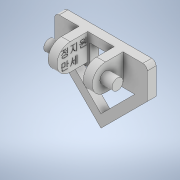
# Autodesk Inventor part: 02-2
Saved by Autodesk Inventor 2022 (Build 260153000, 153)
## iProperties
Created: 2021-09-12
Part Number: 02-2
Material: 일반
Document SubType Name: Modeling
Designer: 서울공업고등학교
Density: 1 g/cm^3
Appearance: 기본값
Author: 서울공업고등학교
Autodesk Inventor part; units mm, degrees
ref_plane "XZ Plane" through (0, 0, 0) normal (0, 1, 0) x (-1, 0, 0)
ref_plane "XY Plane" through (0, 0, 0) normal (0, 0, 1) x (1, 0, 0)
sketch "스케치1" plane through (0, 0, 0) normal (0, 0, 1) x (1, 0, 0)
  line L0 (0, 0) -> (0, 50)
  line L1 (0, 0) -> (50, 0) construction
  line L2 (0, 0) -> (-21, 21)
  line L3 (-21, 21) -> (-21, 35)
  line L4 (-21, 35) -> (0, 35)
  line L5 (0, 5.6569) -> (-15.3431, 21)
  line L6 (-15.3431, 21) -> (-5, 21)
  line L7 (-5, 21) -> (-5, 31)
  line L8 (-5, 31) -> (0, 31)
  line L9 (0, 0) -> (21, 21)
  line L10 (21, 21) -> (21, 35)
  line L11 (21, 35) -> (0, 35)
  line L12 (0, 5.6569) -> (15.3431, 21)
  line L13 (15.3431, 21) -> (5, 21)
  line L14 (5, 21) -> (5, 31)
  line L15 (5, 31) -> (0, 31)
  dimension "d0" = 50
  dimension "d2" = 35
  dimension "d3" = 45
  dimension "d4" = 4
  dimension "d5" = 10
  dimension "d6" = 42
  dimension "d7" = 10
  dimension "d8" = 4
  constraints: 32 end point, 5 symmetric about line, 4 perpendicular, 3 point on line, 2 parallel, 2 vertical, 1 horizontal
  measures "d0" distance of L0.start L0.end
  measures "d2" distance from line of L4 L0.start
  measures "d3" angle of L0 L2
  measures "d4" distance between parallel lines of L4 L8
  measures "d5" distance between parallel lines of L6 L8
  measures "d6" diameter of L3 L0
  measures "d7" diameter of L7 L0
  measures "d8" distance between parallel lines of L2 L5
extrude "돌출1" add sketch "스케치1" against normal blind 4 contours L2 L3 L4 L0 L8 L7 L6 L5 | L0 L12 L13 L14 L15 L11 L10 L9
ref_plane "작업 평면1" through (6, 0, 0) normal (1, 0, 0) x (0, 1, 0)
sketch "스케치2" plane through (6, 0, 0) normal (1, 0, 0) x (0, 1, 0)
  arc A0 (35, 8) -> (23, 8) centre (29, 8) ccw
  circle A1 centre (29, 8) radius 2.5
  line L0 (35, 0) -> (21, 0) projected
  line L1 (35, 0) -> (35, 8)
  line L2 (23, 8) -> (23, 0)
  line L3 (21, -4) -> (35, -4) projected
  point P0 (0, 0)
  dimension "d12" = 12
  dimension "d13" = 5
  dimension "d14" = 12
  dimension "d15" = 18
  dimension "d16" = 12
  constraints: 4 end point, 3 point on circle, 2 centre point, 2 point on line, 1 coincident, 1 parallel, 1 tangent, 1 vertical
  measures "d12" diameter of A0
  measures "d13" diameter of A1
  measures "d14" distance from line of L3 A0.centre
  measures "d16" distance between parallel lines of L2 L1
extrude "돌출2" add sketch "스케치2" along normal blind 4
extrude "돌출3" add sketch "스케치2" along normal blind 9.5 contours A1
mirror "미러1" about plane through (0, 0, 0) normal (1, 0, 0) of "돌출2", "돌출3"
fillet "모깎기1" radius 2 2 edges at (21, 35, -2) (-21, 35, -2)
sketch "스케치3" plane through (-6, 29, 8) normal (1, 0, 0) x (0, 0, -1)
  line L0 (-4.519, 4.2774) -> (7.7198, 4.2774) construction
  line L1 (7.7198, 4.2774) -> (7.7198, -3.1581) construction
  line L2 (7.7198, -3.1581) -> (-4.519, -3.1581) construction
  line L3 (-4.519, -3.1581) -> (-4.519, 4.2774) construction
  spline S0 degree 2 poles (-2.422, 2.0914) (-3.0938, 2.0914) (-3.452, 1.9062) knots 0 0 0 1 1 1
  spline S1 degree 2 poles (-3.452, 1.9062) (-3.7706, 1.7432) (-3.7706, 1.4616) knots 0 0 0 1 1 1
  spline S2 degree 2 poles (-3.7706, 1.4616) (-3.7706, 1.1899) (-3.452, 1.0268) knots 0 0 0 1 1 1
  spline S3 degree 2 poles (-3.452, 1.0268) (-3.0938, 0.8416) (-2.422, 0.8416) knots 0 0 0 1 1 1
  spline S4 degree 2 poles (-2.422, 0.8416) (-1.7526, 0.8416) (-1.3994, 1.0268) knots 0 0 0 1 1 1
  spline S5 degree 2 poles (-1.3994, 1.0268) (-1.0758, 1.1899) (-1.0758, 1.4616) knots 0 0 0 1 1 1
  spline S6 degree 2 poles (-1.0758, 1.4616) (-1.0758, 1.7432) (-1.3994, 1.9062) knots 0 0 0 1 1 1
  spline S7 degree 2 poles (-1.3994, 1.9062) (-1.7526, 2.0914) (-2.422, 2.0914) knots 0 0 0 1 1 1
  spline S8 degree 2 poles (-2.422, 1.879) (-1.8662, 1.879) (-1.5797, 1.7654) knots 0 0 0 1 1 1
  spline S9 degree 2 poles (-1.5797, 1.7654) (-1.3129, 1.6542) (-1.3129, 1.4616) knots 0 0 0 1 1 1
  spline S10 degree 2 poles (-1.3129, 1.4616) (-1.3129, 1.2763) (-1.5797, 1.1701) knots 0 0 0 1 1 1
  spline S11 degree 2 poles (-1.5797, 1.1701) (-1.8662, 1.0515) (-2.422, 1.0515) knots 0 0 0 1 1 1
  spline S12 degree 2 poles (-2.422, 1.0515) (-2.9851, 1.0515) (-3.2717, 1.1701) knots 0 0 0 1 1 1
  spline S13 degree 2 poles (-3.2717, 1.1701) (-3.5335, 1.2763) (-3.5335, 1.4616) knots 0 0 0 1 1 1
  spline S14 degree 2 poles (-3.5335, 1.4616) (-3.5335, 1.6542) (-3.2717, 1.7654) knots 0 0 0 1 1 1
  spline S15 degree 2 poles (-3.2717, 1.7654) (-2.9851, 1.879) (-2.422, 1.879) knots 0 0 0 1 1 1
  line L4 (-1.9774, 4.1786) -> (-3.8348, 4.1786)
  spline S16 degree 2 poles (-3.8348, 4.1786) (-3.9509, 4.1786) (-3.9509, 4.0748) knots 0 0 0 1 1 1
  spline S17 degree 2 poles (-3.9509, 4.0748) (-3.9559, 3.9686) (-3.8398, 3.9686) knots 0 0 0 1 1 1
  line L5 (-3.8398, 3.9686) -> (-3.0296, 3.9686)
  line L6 (-3.0296, 3.9686) -> (-3.0296, 3.8328)
  spline S18 degree 2 poles (-3.0296, 3.8328) (-3.0296, 3.403) (-3.3112, 3.0967) knots 0 0 0 1 1 1
  spline S19 degree 2 poles (-3.3112, 3.0967) (-3.5458, 2.8423) (-3.983, 2.662) knots 0 0 0 1 1 1
  spline S20 degree 2 poles (-3.983, 2.662) (-4.0374, 2.6422) (-4.0522, 2.5978) knots 0 0 0 1 1 1
  spline S21 degree 2 poles (-4.0522, 2.5978) (-4.0645, 2.5558) (-4.0448, 2.5138) knots 0 0 0 1 1 1
  spline S22 degree 2 poles (-4.0448, 2.5138) (-4.0201, 2.4693) (-3.9781, 2.4545) knots 0 0 0 1 1 1
  spline S23 degree 2 poles (-3.9781, 2.4545) (-3.9336, 2.4323) (-3.8818, 2.4496) knots 0 0 0 1 1 1
  spline S24 degree 2 poles (-3.8818, 2.4496) (-3.5137, 2.5928) (-3.2544, 2.8324) knots 0 0 0 1 1 1
  spline S25 degree 2 poles (-3.2544, 2.8324) (-3.0049, 3.0696) (-2.911, 3.3437) knots 0 0 0 1 1 1
  spline S26 degree 2 poles (-2.911, 3.3437) (-2.8419, 3.1017) (-2.5578, 2.8547) knots 0 0 0 1 1 1
  spline S27 degree 2 poles (-2.5578, 2.8547) (-2.296, 2.6299) (-1.9601, 2.4866) knots 0 0 0 1 1 1
  spline S28 degree 2 poles (-1.9601, 2.4866) (-1.9033, 2.4619) (-1.8489, 2.4792) knots 0 0 0 1 1 1
  spline S29 degree 2 poles (-1.8489, 2.4792) (-1.802, 2.4965) (-1.7773, 2.541) knots 0 0 0 1 1 1
  spline S30 degree 2 poles (-1.7773, 2.541) (-1.7551, 2.5854) (-1.7674, 2.6299) knots 0 0 0 1 1 1
  spline S31 degree 2 poles (-1.7674, 2.6299) (-1.7847, 2.6768) (-1.8391, 2.6966) knots 0 0 0 1 1 1
  spline S32 degree 2 poles (-1.8391, 2.6966) (-2.2466, 2.8596) (-2.4837, 3.1066) knots 0 0 0 1 1 1
  spline S33 degree 2 poles (-2.4837, 3.1066) (-2.7875, 3.4154) (-2.7875, 3.8427) knots 0 0 0 1 1 1
  line L7 (-2.7875, 3.8427) -> (-2.7875, 3.9686)
  line L8 (-2.7875, 3.9686) -> (-1.9774, 3.9686)
  spline S34 degree 2 poles (-1.9774, 3.9686) (-1.8736, 3.9686) (-1.8736, 4.0748) knots 0 0 0 1 1 1
  spline S35 degree 2 poles (-1.8736, 4.0748) (-1.8736, 4.1786) (-1.9774, 4.1786) knots 0 0 0 1 1 1
  line L9 (-1.1055, 2.2866) -> (-1.1055, 4.1588)
  spline S36 degree 2 poles (-1.1055, 4.1588) (-1.1055, 4.2156) (-1.145, 4.2478) knots 0 0 0 1 1 1
  spline S37 degree 2 poles (-1.145, 4.2478) (-1.1796, 4.2774) (-1.2265, 4.2774) knots 0 0 0 1 1 1
  spline S38 degree 2 poles (-1.2265, 4.2774) (-1.2808, 4.2774) (-1.3129, 4.2453) knots 0 0 0 1 1 1
  spline S39 degree 2 poles (-1.3129, 4.2453) (-1.35, 4.2107) (-1.35, 4.1539) knots 0 0 0 1 1 1
  line L10 (-1.35, 4.1539) -> (-1.35, 3.4425)
  line L11 (-1.35, 3.4425) -> (-2.0515, 3.4425)
  spline S40 degree 2 poles (-2.0515, 3.4425) (-2.1083, 3.4425) (-2.1355, 3.4129) knots 0 0 0 1 1 1
  spline S41 degree 2 poles (-2.1355, 3.4129) (-2.1651, 3.3808) (-2.1651, 3.3388) knots 0 0 0 1 1 1
  spline S42 degree 2 poles (-2.1651, 3.3388) (-2.1602, 3.2993) (-2.128, 3.2647) knots 0 0 0 1 1 1
  spline S43 degree 2 poles (-2.128, 3.2647) (-2.091, 3.2326) (-2.0292, 3.2326) knots 0 0 0 1 1 1
  line L12 (-2.0292, 3.2326) -> (-1.35, 3.2326)
  line L13 (-1.35, 3.2326) -> (-1.35, 2.2866)
  spline S44 degree 2 poles (-1.35, 2.2866) (-1.35, 2.2248) (-1.3129, 2.1878) knots 0 0 0 1 1 1
  spline S45 degree 2 poles (-1.3129, 2.1878) (-1.2808, 2.1556) (-1.2265, 2.1556) knots 0 0 0 1 1 1
  spline S46 degree 2 poles (-1.2265, 2.1556) (-1.1796, 2.1556) (-1.145, 2.1878) knots 0 0 0 1 1 1
  spline S47 degree 2 poles (-1.145, 2.1878) (-1.1055, 2.2248) (-1.1055, 2.2866) knots 0 0 0 1 1 1
  line L14 (2.2142, 4.149) -> (0.3568, 4.149)
  spline S48 degree 2 poles (0.3568, 4.149) (0.2407, 4.149) (0.2407, 4.0452) knots 0 0 0 1 1 1
  spline S49 degree 2 poles (0.2407, 4.0452) (0.2358, 3.939) (0.3519, 3.939) knots 0 0 0 1 1 1
  line L15 (0.3519, 3.939) -> (1.162, 3.939)
  line L16 (1.162, 3.939) -> (1.162, 3.2721)
  spline S50 degree 2 poles (1.162, 3.2721) (1.162, 2.6324) (0.8878, 2.1062) knots 0 0 0 1 1 1
  spline S51 degree 2 poles (0.8878, 2.1062) (0.626, 1.59) (0.2135, 1.3776) knots 0 0 0 1 1 1
  spline S52 degree 2 poles (0.2135, 1.3776) (0.1592, 1.3529) (0.1419, 1.3035) knots 0 0 0 1 1 1
  spline S53 degree 2 poles (0.1419, 1.3035) (0.1296, 1.259) (0.1543, 1.2121) knots 0 0 0 1 1 1
  spline S54 degree 2 poles (0.1543, 1.2121) (0.1765, 1.1726) (0.216, 1.1553) knots 0 0 0 1 1 1
  spline S55 degree 2 poles (0.216, 1.1553) (0.2605, 1.1355) (0.3099, 1.1602) knots 0 0 0 1 1 1
  spline S56 degree 2 poles (0.3099, 1.1602) (0.6557, 1.3307) (0.9298, 1.7357) knots 0 0 0 1 1 1
  spline S57 degree 2 poles (0.9298, 1.7357) (1.1991, 2.1334) (1.2806, 2.5632) knots 0 0 0 1 1 1
  spline S58 degree 2 poles (1.2806, 2.5632) (1.3497, 2.1458) (1.6289, 1.7357) knots 0 0 0 1 1 1
  spline S59 degree 2 poles (1.6289, 1.7357) (1.908, 1.3356) (2.234, 1.1602) knots 0 0 0 1 1 1
  spline S60 degree 2 poles (2.234, 1.1602) (2.2958, 1.1257) (2.3501, 1.1429) knots 0 0 0 1 1 1
  spline S61 degree 2 poles (2.3501, 1.1429) (2.3995, 1.1553) (2.4242, 1.1998) knots 0 0 0 1 1 1
  spline S62 degree 2 poles (2.4242, 1.1998) (2.444, 1.2417) (2.4316, 1.2911) knots 0 0 0 1 1 1
  spline S63 degree 2 poles (2.4316, 1.2911) (2.4193, 1.3405) (2.3649, 1.3677) knots 0 0 0 1 1 1
  spline S64 degree 2 poles (2.3649, 1.3677) (1.9351, 1.6048) (1.6733, 2.1137) knots 0 0 0 1 1 1
  spline S65 degree 2 poles (1.6733, 2.1137) (1.4041, 2.6373) (1.4041, 3.277) knots 0 0 0 1 1 1
  line L17 (1.4041, 3.277) -> (1.4041, 3.939)
  line L18 (1.4041, 3.939) -> (2.2142, 3.939)
  spline S66 degree 2 poles (2.2142, 3.939) (2.318, 3.939) (2.318, 4.0452) knots 0 0 0 1 1 1
  spline S67 degree 2 poles (2.318, 4.0452) (2.318, 4.149) (2.2142, 4.149) knots 0 0 0 1 1 1
  line L19 (3.0862, 0.975) -> (3.0862, 4.1613)
  spline S68 degree 2 poles (3.0862, 4.1613) (3.0862, 4.2156) (3.0466, 4.2478) knots 0 0 0 1 1 1
  spline S69 degree 2 poles (3.0466, 4.2478) (3.0121, 4.2725) (2.9651, 4.2725) knots 0 0 0 1 1 1
  spline S70 degree 2 poles (2.9651, 4.2725) (2.9108, 4.2725) (2.8787, 4.2478) knots 0 0 0 1 1 1
  spline S71 degree 2 poles (2.8787, 4.2478) (2.8416, 4.2156) (2.8416, 4.1613) knots 0 0 0 1 1 1
  line L20 (2.8416, 4.1613) -> (2.8416, 0.975)
  spline S72 degree 2 poles (2.8416, 0.975) (2.8416, 0.9182) (2.8787, 0.8811) knots 0 0 0 1 1 1
  spline S73 degree 2 poles (2.8787, 0.8811) (2.9108, 0.849) (2.9651, 0.849) knots 0 0 0 1 1 1
  spline S74 degree 2 poles (2.9651, 0.849) (3.0121, 0.849) (3.0466, 0.8811) knots 0 0 0 1 1 1
  spline S75 degree 2 poles (3.0466, 0.8811) (3.0862, 0.9182) (3.0862, 0.975) knots 0 0 0 1 1 1
  spline S76 degree 2 poles (5.5068, 4.1934) (4.9807, 4.1934) (4.6892, 4.0082) knots 0 0 0 1 1 1
  spline S77 degree 2 poles (4.6892, 4.0082) (4.4323, 3.8451) (4.4323, 3.5957) knots 0 0 0 1 1 1
  spline S78 degree 2 poles (4.4323, 3.5957) (4.4323, 3.3511) (4.6892, 3.1881) knots 0 0 0 1 1 1
  spline S79 degree 2 poles (4.6892, 3.1881) (4.9807, 3.0029) (5.5068, 3.0029) knots 0 0 0 1 1 1
  spline S80 degree 2 poles (5.5068, 3.0029) (6.0255, 3.0029) (6.3169, 3.1881) knots 0 0 0 1 1 1
  spline S81 degree 2 poles (6.3169, 3.1881) (6.5788, 3.3511) (6.5788, 3.5957) knots 0 0 0 1 1 1
  spline S82 degree 2 poles (6.5788, 3.5957) (6.5788, 3.8451) (6.3169, 4.0082) knots 0 0 0 1 1 1
  spline S83 degree 2 poles (6.3169, 4.0082) (6.0255, 4.1934) (5.5068, 4.1934) knots 0 0 0 1 1 1
  spline S84 degree 2 poles (5.5068, 3.9835) (5.9193, 3.9835) (6.1391, 3.8649) knots 0 0 0 1 1 1
  spline S85 degree 2 poles (6.1391, 3.8649) (6.3367, 3.7587) (6.3367, 3.5957) knots 0 0 0 1 1 1
  spline S86 degree 2 poles (6.3367, 3.5957) (6.3367, 3.4376) (6.1391, 3.3314) knots 0 0 0 1 1 1
  spline S87 degree 2 poles (6.1391, 3.3314) (5.9193, 3.2128) (5.5068, 3.2128) knots 0 0 0 1 1 1
  spline S88 degree 2 poles (5.5068, 3.2128) (5.0869, 3.2128) (4.867, 3.3314) knots 0 0 0 1 1 1
  spline S89 degree 2 poles (4.867, 3.3314) (4.6744, 3.4376) (4.6744, 3.5957) knots 0 0 0 1 1 1
  spline S90 degree 2 poles (4.6744, 3.5957) (4.6744, 3.7587) (4.867, 3.8649) knots 0 0 0 1 1 1
  spline S91 degree 2 poles (4.867, 3.8649) (5.0869, 3.9835) (5.5068, 3.9835) knots 0 0 0 1 1 1
  line L21 (7.2778, 1.8444) -> (7.2778, 4.1662)
  spline S92 degree 2 poles (7.2778, 4.1662) (7.2778, 4.2206) (7.2383, 4.2478) knots 0 0 0 1 1 1
  spline S93 degree 2 poles (7.2383, 4.2478) (7.2037, 4.2774) (7.1567, 4.2774) knots 0 0 0 1 1 1
  spline S94 degree 2 poles (7.1567, 4.2774) (7.1024, 4.2774) (7.0703, 4.2478) knots 0 0 0 1 1 1
  spline S95 degree 2 poles (7.0703, 4.2478) (7.0332, 4.2156) (7.0332, 4.1638) knots 0 0 0 1 1 1
  line L22 (7.0332, 4.1638) -> (7.0332, 2.3656)
  line L23 (7.0332, 2.3656) -> (6.2206, 2.3656)
  spline S96 degree 2 poles (6.2206, 2.3656) (6.1638, 2.3656) (6.1317, 2.336) knots 0 0 0 1 1 1
  spline S97 degree 2 poles (6.1317, 2.336) (6.1021, 2.3088) (6.107, 2.2643) knots 0 0 0 1 1 1
  spline S98 degree 2 poles (6.107, 2.2643) (6.107, 2.2223) (6.144, 2.1927) knots 0 0 0 1 1 1
  spline S99 degree 2 poles (6.144, 2.1927) (6.1811, 2.1606) (6.2453, 2.1606) knots 0 0 0 1 1 1
  line L24 (6.2453, 2.1606) -> (7.0332, 2.1606)
  line L25 (7.0332, 2.1606) -> (7.0332, 1.8444)
  spline S100 degree 2 poles (7.0332, 1.8444) (7.0332, 1.7876) (7.0703, 1.7506) knots 0 0 0 1 1 1
  spline S101 degree 2 poles (7.0703, 1.7506) (7.1024, 1.7209) (7.1567, 1.7209) knots 0 0 0 1 1 1
  spline S102 degree 2 poles (7.1567, 1.7209) (7.2037, 1.7209) (7.2383, 1.7506) knots 0 0 0 1 1 1
  spline S103 degree 2 poles (7.2383, 1.7506) (7.2778, 1.7876) (7.2778, 1.8444) knots 0 0 0 1 1 1
  spline S104 degree 2 poles (4.8868, 1.8271) (4.8868, 1.8864) (4.8473, 1.9185) knots 0 0 0 1 1 1
  spline S105 degree 2 poles (4.8473, 1.9185) (4.8127, 1.9506) (4.7658, 1.9506) knots 0 0 0 1 1 1
  spline S106 degree 2 poles (4.7658, 1.9506) (4.7114, 1.9506) (4.6793, 1.9185) knots 0 0 0 1 1 1
  spline S107 degree 2 poles (4.6793, 1.9185) (4.6423, 1.8839) (4.6423, 1.8271) knots 0 0 0 1 1 1
  line L26 (4.6423, 1.8271) -> (4.6423, 1.3109)
  spline S108 degree 2 poles (4.6423, 1.3109) (4.6423, 1.1528) (4.7534, 1.0491) knots 0 0 0 1 1 1
  spline S109 degree 2 poles (4.7534, 1.0491) (4.8646, 0.9478) (5.0301, 0.9478) knots 0 0 0 1 1 1
  line L27 (5.0301, 0.9478) -> (7.3074, 0.9478)
  spline S110 degree 2 poles (7.3074, 0.9478) (7.4136, 0.9478) (7.4136, 1.054) knots 0 0 0 1 1 1
  spline S111 degree 2 poles (7.4136, 1.054) (7.4136, 1.1578) (7.3074, 1.1578) knots 0 0 0 1 1 1
  line L28 (7.3074, 1.1578) -> (5.0869, 1.1578)
  spline S112 degree 2 poles (5.0869, 1.1578) (4.9683, 1.1578) (4.9288, 1.1948) knots 0 0 0 1 1 1
  spline S113 degree 2 poles (4.9288, 1.1948) (4.8868, 1.2343) (4.8868, 1.3455) knots 0 0 0 1 1 1
  line L29 (4.8868, 1.3455) -> (4.8868, 1.8271)
  line L30 (5.366, 2.5286) -> (5.366, 2.3483)
  spline S114 degree 2 poles (5.366, 2.3483) (5.366, 2.2372) (5.3413, 2.1482) knots 0 0 0 1 1 1
  spline S115 degree 2 poles (5.3413, 2.1482) (5.3166, 2.0568) (5.2795, 1.9926) knots 0 0 0 1 1 1
  spline S116 degree 2 poles (5.2795, 1.9926) (5.2104, 1.9012) (5.2919, 1.842) knots 0 0 0 1 1 1
  spline S117 degree 2 poles (5.2919, 1.842) (5.3734, 1.7753) (5.4475, 1.8568) knots 0 0 0 1 1 1
  spline S118 degree 2 poles (5.4475, 1.8568) (5.5167, 1.9432) (5.5611, 2.0815) knots 0 0 0 1 1 1
  spline S119 degree 2 poles (5.5611, 2.0815) (5.6105, 2.2248) (5.6105, 2.3779) knots 0 0 0 1 1 1
  line L31 (5.6105, 2.3779) -> (5.6105, 2.541)
  line L32 (5.6105, 2.541) -> (6.6183, 2.5706)
  spline S120 degree 2 poles (6.6183, 2.5706) (6.6677, 2.5755) (6.6998, 2.6126) knots 0 0 0 1 1 1
  spline S121 degree 2 poles (6.6998, 2.6126) (6.7245, 2.6398) (6.7245, 2.6818) knots 0 0 0 1 1 1
  spline S122 degree 2 poles (6.7245, 2.6818) (6.7196, 2.7262) (6.6874, 2.7509) knots 0 0 0 1 1 1
  spline S123 degree 2 poles (6.6874, 2.7509) (6.6504, 2.7781) (6.5936, 2.7707) knots 0 0 0 1 1 1
  spline S124 degree 2 poles (6.5936, 2.7707) (6.2132, 2.7509) (5.5265, 2.7336) knots 0 0 0 1 1 1
  spline S125 degree 2 poles (5.5265, 2.7336) (4.8819, 2.7163) (4.3187, 2.7163) knots 0 0 0 1 1 1
  spline S126 degree 2 poles (4.3187, 2.7163) (4.2125, 2.7163) (4.2075, 2.6175) knots 0 0 0 1 1 1
  spline S127 degree 2 poles (4.2075, 2.6175) (4.2026, 2.5163) (4.3063, 2.5163) knots 0 0 0 1 1 1
  line L33 (4.3063, 2.5163) -> (5.366, 2.5286)
  line L34 (-2.6171, -0.8695) -> (-3.5878, -0.8695)
  spline S128 degree 2 poles (-3.5878, -0.8695) (-3.7533, -0.8695) (-3.8571, -0.9757) knots 0 0 0 1 1 1
  spline S129 degree 2 poles (-3.8571, -0.9757) (-3.9509, -1.0745) (-3.9509, -1.2227) knots 0 0 0 1 1 1
  line L35 (-3.9509, -1.2227) -> (-3.9509, -2.3565)
  spline S130 degree 2 poles (-3.9509, -2.3565) (-3.9509, -2.5047) (-3.862, -2.5985) knots 0 0 0 1 1 1
  spline S131 degree 2 poles (-3.862, -2.5985) (-3.7657, -2.6924) (-3.615, -2.6924) knots 0 0 0 1 1 1
  line L36 (-3.615, -2.6924) -> (-2.6048, -2.6924)
  spline S132 degree 2 poles (-2.6048, -2.6924) (-2.4368, -2.6924) (-2.3331, -2.6035) knots 0 0 0 1 1 1
  spline S133 degree 2 poles (-2.3331, -2.6035) (-2.2318, -2.5121) (-2.2318, -2.3515) knots 0 0 0 1 1 1
  line L37 (-2.2318, -2.3515) -> (-2.2318, -1.1931)
  spline S134 degree 2 poles (-2.2318, -1.1931) (-2.2318, -1.0548) (-2.338, -0.9634) knots 0 0 0 1 1 1
  spline S135 degree 2 poles (-2.338, -0.9634) (-2.4442, -0.8695) (-2.6171, -0.8695) knots 0 0 0 1 1 1
  line L38 (-2.4689, -1.2548) -> (-2.4689, -2.3268)
  spline S136 degree 2 poles (-2.4689, -2.3268) (-2.4689, -2.4157) (-2.5134, -2.4528) knots 0 0 0 1 1 1
  spline S137 degree 2 poles (-2.5134, -2.4528) (-2.5554, -2.4824) (-2.6542, -2.4824) knots 0 0 0 1 1 1
  line L39 (-2.6542, -2.4824) -> (-3.5285, -2.4824)
  spline S138 degree 2 poles (-3.5285, -2.4824) (-3.6323, -2.4824) (-3.6669, -2.4503) knots 0 0 0 1 1 1
  spline S139 degree 2 poles (-3.6669, -2.4503) (-3.7089, -2.4157) (-3.7089, -2.3268) knots 0 0 0 1 1 1
  line L40 (-3.7089, -2.3268) -> (-3.7089, -1.2721)
  spline S140 degree 2 poles (-3.7089, -1.2721) (-3.7089, -1.1659) (-3.6718, -1.1239) knots 0 0 0 1 1 1
  spline S141 degree 2 poles (-3.6718, -1.1239) (-3.6323, -1.0795) (-3.5335, -1.0795) knots 0 0 0 1 1 1
  line L41 (-3.5335, -1.0795) -> (-2.6616, -1.0795)
  spline S142 degree 2 poles (-2.6616, -1.0795) (-2.5554, -1.0795) (-2.5109, -1.1239) knots 0 0 0 1 1 1
  spline S143 degree 2 poles (-2.5109, -1.1239) (-2.4689, -1.1659) (-2.4689, -1.2548) knots 0 0 0 1 1 1
  spline S144 degree 2 poles (-3.5063, -3.1567) (-3.5063, -3.0876) (-3.5483, -3.0505) knots 0 0 0 1 1 1
  spline S145 degree 2 poles (-3.5483, -3.0505) (-3.5804, -3.0135) (-3.6298, -3.0135) knots 0 0 0 1 1 1
  spline S146 degree 2 poles (-3.6298, -3.0135) (-3.6792, -3.0135) (-3.7113, -3.0505) knots 0 0 0 1 1 1
  spline S147 degree 2 poles (-3.7113, -3.0505) (-3.7484, -3.0876) (-3.7484, -3.1567) knots 0 0 0 1 1 1
  line L42 (-3.7484, -3.1567) -> (-3.7484, -3.6977)
  spline S148 degree 2 poles (-3.7484, -3.6977) (-3.7484, -3.8706) (-3.6471, -3.9694) knots 0 0 0 1 1 1
  spline S149 degree 2 poles (-3.6471, -3.9694) (-3.536, -4.0706) (-3.3433, -4.0706) knots 0 0 0 1 1 1
  line L43 (-3.3433, -4.0706) -> (-1.224, -4.0706)
  spline S150 degree 2 poles (-1.224, -4.0706) (-1.1178, -4.0706) (-1.1178, -3.9644) knots 0 0 0 1 1 1
  spline S151 degree 2 poles (-1.1178, -3.9644) (-1.1178, -3.8607) (-1.224, -3.8607) knots 0 0 0 1 1 1
  line L44 (-1.224, -3.8607) -> (-3.3112, -3.8607)
  spline S152 degree 2 poles (-3.3112, -3.8607) (-3.4248, -3.8607) (-3.4643, -3.8236) knots 0 0 0 1 1 1
  spline S153 degree 2 poles (-3.4643, -3.8236) (-3.5063, -3.7841) (-3.5063, -3.673) knots 0 0 0 1 1 1
  line L45 (-3.5063, -3.673) -> (-3.5063, -3.1567)
  line L46 (-1.224, -1.9785) -> (-1.224, -0.8522)
  spline S154 degree 2 poles (-1.224, -0.8522) (-1.224, -0.7411) (-1.3475, -0.7411) knots 0 0 0 1 1 1
  spline S155 degree 2 poles (-1.3475, -0.7411) (-1.4661, -0.7411) (-1.4661, -0.8522) knots 0 0 0 1 1 1
  line L47 (-1.4661, -0.8522) -> (-1.4661, -3.1197)
  spline S156 degree 2 poles (-1.4661, -3.1197) (-1.4661, -3.1765) (-1.429, -3.2111) knots 0 0 0 1 1 1
  spline S157 degree 2 poles (-1.429, -3.2111) (-1.3969, -3.2432) (-1.3475, -3.2432) knots 0 0 0 1 1 1
  spline S158 degree 2 poles (-1.3475, -3.2432) (-1.2981, -3.2432) (-1.266, -3.2111) knots 0 0 0 1 1 1
  spline S159 degree 2 poles (-1.266, -3.2111) (-1.224, -3.179) (-1.224, -3.1197) knots 0 0 0 1 1 1
  line L48 (-1.224, -3.1197) -> (-1.224, -2.1885)
  line L49 (-1.224, -2.1885) -> (-0.7769, -2.1885)
  spline S160 degree 2 poles (-0.7769, -2.1885) (-0.6707, -2.1885) (-0.6707, -2.0823) knots 0 0 0 1 1 1
  spline S161 degree 2 poles (-0.6707, -2.0823) (-0.6707, -1.9785) (-0.7769, -1.9785) knots 0 0 0 1 1 1
  line L50 (-0.7769, -1.9785) -> (-1.224, -1.9785)
  spline S162 degree 2 poles (0.9002, -0.9609) (0.9002, -1.8106) (0.668, -2.5639) knots 0 0 0 1 1 1
  spline S163 degree 2 poles (0.668, -2.5639) (0.463, -3.2284) (0.1345, -3.6507) knots 0 0 0 1 1 1
  spline S164 degree 2 poles (0.1345, -3.6507) (0.095, -3.7026) (0.0974, -3.752) knots 0 0 0 1 1 1
  spline S165 degree 2 poles (0.0974, -3.752) (0.0974, -3.794) (0.1345, -3.8162) knots 0 0 0 1 1 1
  spline S166 degree 2 poles (0.1345, -3.8162) (0.1666, -3.8409) (0.2135, -3.8335) knots 0 0 0 1 1 1
  spline S167 degree 2 poles (0.2135, -3.8335) (0.2605, -3.8212) (0.2975, -3.7817) knots 0 0 0 1 1 1
  spline S168 degree 2 poles (0.2975, -3.7817) (0.5371, -3.4778) (0.7026, -3.0999) knots 0 0 0 1 1 1
  spline S169 degree 2 poles (0.7026, -3.0999) (0.8434, -2.7862) (0.9447, -2.4059) knots 0 0 0 1 1 1
  spline S170 degree 2 poles (0.9447, -2.4059) (1.1423, -2.6998) (1.3226, -3.0308) knots 0 0 0 1 1 1
  spline S171 degree 2 poles (1.3226, -3.0308) (1.4905, -3.3469) (1.6536, -3.7199) knots 0 0 0 1 1 1
  spline S172 degree 2 poles (1.6536, -3.7199) (1.6783, -3.7767) (1.7227, -3.8014) knots 0 0 0 1 1 1
  spline S173 degree 2 poles (1.7227, -3.8014) (1.7696, -3.8212) (1.8092, -3.8039) knots 0 0 0 1 1 1
  spline S174 degree 2 poles (1.8092, -3.8039) (1.8512, -3.7891) (1.866, -3.7446) knots 0 0 0 1 1 1
  spline S175 degree 2 poles (1.866, -3.7446) (1.8833, -3.6952) (1.8536, -3.6334) knots 0 0 0 1 1 1
  spline S176 degree 2 poles (1.8536, -3.6334) (1.6955, -3.2432) (1.4856, -2.8801) knots 0 0 0 1 1 1
  spline S177 degree 2 poles (1.4856, -2.8801) (1.2905, -2.5368) (1.0113, -2.1391) knots 0 0 0 1 1 1
  spline S178 degree 2 poles (1.0113, -2.1391) (1.0756, -1.7538) (1.1101, -1.4524) knots 0 0 0 1 1 1
  spline S179 degree 2 poles (1.1101, -1.4524) (1.1423, -1.1684) (1.1423, -0.9609) knots 0 0 0 1 1 1
  spline S180 degree 2 poles (1.1423, -0.9609) (1.1423, -0.8991) (1.1003, -0.867) knots 0 0 0 1 1 1
  spline S181 degree 2 poles (1.1003, -0.867) (1.0682, -0.8374) (1.0188, -0.8374) knots 0 0 0 1 1 1
  spline S182 degree 2 poles (1.0188, -0.8374) (0.9694, -0.8374) (0.9372, -0.867) knots 0 0 0 1 1 1
  spline S183 degree 2 poles (0.9372, -0.867) (0.9002, -0.8991) (0.9002, -0.9609) knots 0 0 0 1 1 1
  line L51 (2.4415, -4.0435) -> (2.4415, -0.8522)
  spline S184 degree 2 poles (2.4415, -0.8522) (2.4415, -0.7979) (2.3995, -0.7707) knots 0 0 0 1 1 1
  spline S185 degree 2 poles (2.3995, -0.7707) (2.3674, -0.7411) (2.318, -0.7411) knots 0 0 0 1 1 1
  spline S186 degree 2 poles (2.318, -0.7411) (2.2686, -0.7411) (2.2365, -0.7707) knots 0 0 0 1 1 1
  spline S187 degree 2 poles (2.2365, -0.7707) (2.1994, -0.8028) (2.1994, -0.8547) knots 0 0 0 1 1 1
  line L52 (2.1994, -0.8547) -> (2.1994, -2.1292)
  line L53 (2.1994, -2.1292) -> (1.4362, -2.1292)
  spline S188 degree 2 poles (1.4362, -2.1292) (1.3794, -2.1292) (1.3473, -2.1589) knots 0 0 0 1 1 1
  spline S189 degree 2 poles (1.3473, -2.1589) (1.3176, -2.191) (1.3226, -2.233) knots 0 0 0 1 1 1
  spline S190 degree 2 poles (1.3226, -2.233) (1.3226, -2.2725) (1.3547, -2.3071) knots 0 0 0 1 1 1
  spline S191 degree 2 poles (1.3547, -2.3071) (1.3917, -2.3392) (1.4584, -2.3392) knots 0 0 0 1 1 1
  line L54 (1.4584, -2.3392) -> (2.1994, -2.3392)
  line L55 (2.1994, -2.3392) -> (2.1994, -4.0435)
  spline S192 degree 2 poles (2.1994, -4.0435) (2.1994, -4.1003) (2.2365, -4.1373) knots 0 0 0 1 1 1
  spline S193 degree 2 poles (2.2365, -4.1373) (2.2686, -4.1694) (2.318, -4.1694) knots 0 0 0 1 1 1
  spline S194 degree 2 poles (2.318, -4.1694) (2.3674, -4.1694) (2.3995, -4.1373) knots 0 0 0 1 1 1
  spline S195 degree 2 poles (2.3995, -4.1373) (2.4415, -4.1003) (2.4415, -4.0435) knots 0 0 0 1 1 1
  line L56 (3.1973, -4.0435) -> (3.1973, -0.8522)
  spline S196 degree 2 poles (3.1973, -0.8522) (3.1973, -0.7979) (3.1553, -0.7707) knots 0 0 0 1 1 1
  spline S197 degree 2 poles (3.1553, -0.7707) (3.1232, -0.7411) (3.0788, -0.7411) knots 0 0 0 1 1 1
  spline S198 degree 2 poles (3.0788, -0.7411) (3.0294, -0.7411) (2.9972, -0.7707) knots 0 0 0 1 1 1
  spline S199 degree 2 poles (2.9972, -0.7707) (2.9602, -0.8028) (2.9602, -0.8547) knots 0 0 0 1 1 1
  line L57 (2.9602, -0.8547) -> (2.9602, -4.0435)
  spline S200 degree 2 poles (2.9602, -4.0435) (2.9602, -4.1003) (2.9972, -4.1373) knots 0 0 0 1 1 1
  spline S201 degree 2 poles (2.9972, -4.1373) (3.0294, -4.1694) (3.0788, -4.1694) knots 0 0 0 1 1 1
  spline S202 degree 2 poles (3.0788, -4.1694) (3.1232, -4.1694) (3.1553, -4.1373) knots 0 0 0 1 1 1
  spline S203 degree 2 poles (3.1553, -4.1373) (3.1973, -4.1003) (3.1973, -4.0435) knots 0 0 0 1 1 1
  point P0 (8, -29)
  constraints: 2 other
extrude "돌출4" cut sketch "스케치3" against normal blind 1
